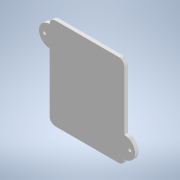
# Autodesk Inventor part: lid_arm
Saved by Autodesk Inventor 2021 (Build 250183000, 183)
## iProperties
Created: 2021-12-14
Part Number: lid_arm
Material: Generic
Document SubType Name: Modeling
Designer: marcin
Density: 1 g/cm^3
Appearance: Default
Author: marcin
Autodesk Inventor part; units mm, degrees
ref_plane "YZ Plane" through (0, 0, 0) normal (1, 0, 0) x (0, 1, 0)
ref_plane "XZ Plane" through (0, 0, 0) normal (0, 1, 0) x (-1, 0, 0)
ref_plane "XY Plane" through (0, 0, 0) normal (0, 0, 1) x (1, 0, 0)
sketch "Sketch3" plane through (0, 0, 0) normal (0, 0, 1) x (1, 0, 0)
  line L0 (-23.255, 22.635) -> (-23.255, -27.435) projected
  line L1 (-18.255, -32.435) -> (-8.145, -32.435) projected
  line L2 (-8.145, -32.435) -> (-8.145, -29.435) projected
  line L3 (-8.145, -29.435) -> (-20.255, -29.435) projected
  line L4 (-20.255, -29.435) -> (-20.255, 42.635) projected
  line L5 (-20.255, 42.635) -> (-8.145, 42.635) projected
  line L6 (-8.145, 42.635) -> (-8.145, 45.635) projected
  line L7 (-8.145, 45.635) -> (-18.255, 45.635) projected
  arc A0 (-23.255, 40.635) -> (-23.255, 22.635) centre (-23.255, 31.635) ccw projected
  circle A1 centre (-27.755, 31.635) radius 1.25 projected
  line L8 (-8.145, 45.635) -> (-18.255, 45.635) projected
  line L9 (-18.255, -32.435) -> (-8.145, -32.435) projected
  line L10 (-8.145, -29.435) -> (7.855, -29.435) projected
  line L11 (-8.145, -32.435) -> (-8.145, -29.435) projected
  line L12 (7.855, -32.435) -> (-8.145, -32.435) projected
  line L13 (7.855, -32.435) -> (7.855, -29.435) projected
  line L14 (7.855, 42.635) -> (-8.145, 42.635) projected
  line L15 (7.855, 45.635) -> (7.855, 42.635) projected
  line L16 (-8.145, 45.635) -> (7.855, 45.635) projected
  line L17 (-8.145, 45.635) -> (-8.145, 42.635) projected
  line L18 (-23.255, 22.635) -> (-23.255, -27.435) projected
  arc A2 (-23.255, -27.435) -> (-18.255, -32.435) centre (-18.255, -27.435) ccw projected
  line L19 (-8.145, -32.435) -> (-8.145, -29.435) projected
  line L20 (-8.145, -29.435) -> (-20.255, -29.435) projected
  line L21 (-20.255, -29.435) -> (-20.255, 42.635) projected
  line L22 (-20.255, 42.635) -> (-8.145, 42.635) projected
  line L23 (-8.145, 42.635) -> (-8.145, 45.635) projected
  arc A3 (-18.255, 45.635) -> (-23.255, 40.635) centre (-18.255, 40.635) ccw projected
  arc A4 (-23.255, 40.635) -> (-23.255, 22.635) centre (-23.255, 31.635) ccw projected
  circle A5 centre (-27.755, 31.635) radius 1.25 projected
  arc A6 (-23.255, -27.435) -> (-18.255, -32.435) centre (-18.255, -27.435) ccw projected
  arc A7 (-18.255, 45.635) -> (-23.255, 40.635) centre (-18.255, 40.635) ccw projected
  line L24 (40.455, -9.435) -> (40.455, 40.635) projected
  arc A8 (40.455, 40.635) -> (35.455, 45.635) centre (35.455, 40.635) ccw projected
  line L25 (35.455, 45.635) -> (7.855, 45.635) projected
  line L26 (7.855, 45.635) -> (7.855, 42.635) projected
  line L27 (7.855, 42.635) -> (37.455, 42.635) projected
  line L28 (37.455, 42.635) -> (37.455, -29.435) projected
  line L29 (37.455, -29.435) -> (7.855, -29.435) projected
  line L30 (7.855, -29.435) -> (7.855, -32.435) projected
  line L31 (7.855, -32.435) -> (35.455, -32.435) projected
  arc A9 (35.455, -32.435) -> (40.455, -27.435) centre (35.455, -27.435) ccw projected
  arc A10 (40.455, -27.435) -> (40.455, -9.435) centre (40.455, -18.435) ccw projected
  circle A11 centre (44.955, -18.435) radius 1.25 projected
  point P0 (0, 0)
extrude "Extrusion3" add sketch "Sketch3" along normal blind 3
sketch "Sketch5" plane through (0, 0, 0) normal (0, 0, -1) x (-1, 0, 0)
  line L0 (20.255, -29.435) -> (20.255, 42.635) projected
  line L1 (8.145, -29.435) -> (20.255, -29.435) projected
  line L2 (-37.455, -29.435) -> (-7.855, -29.435) projected
  line L3 (-37.455, 42.635) -> (-37.455, -29.435) projected
  line L4 (-7.855, 42.635) -> (-37.455, 42.635) projected
  line L5 (20.255, 42.635) -> (8.145, 42.635) projected
  line L6 (-7.855, 42.635) -> (8.145, 42.635)
  line L7 (-7.855, -29.435) -> (8.145, -29.435)
  line L8 (20.055, -29.235) -> (-37.255, -29.235)
  line L9 (-37.255, -29.235) -> (-37.255, 42.435)
  line L10 (-37.255, 42.435) -> (-7.855, 42.435)
  line L11 (-7.855, 42.435) -> (8.145, 42.435)
  line L12 (8.145, 42.435) -> (20.055, 42.435)
  line L13 (20.055, 42.435) -> (20.055, -29.235)
  line L14 (-36.255, -28.235) -> (19.055, -28.235)
  line L15 (19.055, -28.235) -> (19.055, 41.435)
  line L16 (19.055, 41.435) -> (-36.255, 41.435)
  line L17 (-36.255, 41.435) -> (-36.255, -28.235)
  point P0 (0, 0)
  dimension "d8" = 0.2
  dimension "d9" = 1
  constraints: 24 end point, 1 horizontal, 1 parallel, 8 other
  measures "d8" distance between parallel lines of L2 L8
  measures "d9" distance between parallel lines of L8 L14
extrude "Extrusion4" add sketch "Sketch5" along normal blind 2 contours L8 L9 L10 L11 L12 L13
body "Solid2"
